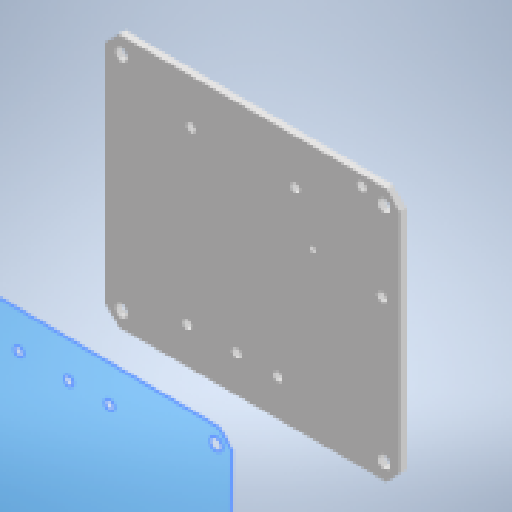
# Autodesk Inventor part: board_rpi
Saved by Autodesk Inventor 2025 (Build 290162000, 162)
## iProperties
Created: 2026-07-21
Part Number: board_rpi
Material: Типовые
Document SubType Name: Modeling
Designer: garin
Density: 1 g/cm^3
Appearance: По умолчанию
Author: garin
Autodesk Inventor part; units mm, degrees
ref_plane "YZ Plane" through (0, 0, 0) normal (1, 0, 0) x (0, 1, 0)
ref_plane "XZ Plane" through (0, 0, 0) normal (0, 1, 0) x (-1, 0, 0)
ref_plane "XY Plane" through (0, 0, 0) normal (0, 0, 1) x (1, 0, 0)
sketch "Эскиз1" plane through (0, 0, 0) normal (0, 0, 1) x (1, 0, 0)
  line L0 (-73.63, -2.23) -> (5.37, -2.23) projected
  arc A0 (5.37, -2.23) -> (8.37, 0.77) centre (5.37, 0.77) ccw projected
  line L1 (8.37, 0.77) -> (8.37, 50.77) projected
  arc A1 (8.37, 50.77) -> (5.37, 53.77) centre (5.37, 50.77) ccw projected
  line L2 (5.37, 53.77) -> (-73.63, 53.77) projected
  arc A2 (-73.63, 53.77) -> (-76.63, 50.77) centre (-73.63, 50.77) ccw projected
  line L3 (-76.63, 50.77) -> (-76.63, 0.77) projected
  arc A3 (-76.63, 0.77) -> (-73.63, -2.23) centre (-73.63, 0.77) ccw projected
  circle A4 centre (4.87, 50.27) radius 1.35 projected
  circle A5 centre (-53.13, 50.27) radius 1.35 projected
  circle A6 centre (0.07, 48.67) radius 0.325 projected
  circle A7 centre (-5.73, 48.67) radius 0.325 projected
  circle A8 centre (-68.88, 49.235) radius 1.65 projected
  circle A9 centre (4.87, 44.27) radius 1.55 projected
  circle A10 centre (-68.88, 37.805) radius 1.65 projected
  circle A11 centre (-53.13, 7.27) radius 1.55 projected
  circle A12 centre (4.87, 1.27) radius 1.35 projected
  circle A13 centre (-53.13, 1.27) radius 1.35 projected
  line L4 (5.37, -2.23) -> (8.37, -2.23) construction
  line L5 (8.37, -2.23) -> (8.37, 0.77) construction
  line L6 (8.37, 0.77) -> (5.37, 0.77) construction
  line L7 (5.37, 0.77) -> (5.37, -2.23) construction
  line L8 (8.37, -2.23) -> (-56.63, -2.23)
  line L9 (-56.63, -2.23) -> (-56.63, 53.77)
  line L10 (-56.63, 53.77) -> (8.37, 53.77)
  line L11 (8.37, 53.77) -> (8.37, -2.23)
  line L12 (8.37, -2.23) -> (-56.63, -2.23)
  line L13 (-56.63, -2.23) -> (-56.63, -13.23)
  line L14 (-56.63, -13.23) -> (8.37, -13.23)
  line L15 (8.37, -13.23) -> (8.37, -2.23)
  line L16 (-56.63, 53.77) -> (8.37, 53.77)
  line L17 (8.37, 53.77) -> (8.37, 61.77)
  line L18 (8.37, 61.77) -> (-56.63, 61.77)
  line L19 (-56.63, 61.77) -> (-56.63, 53.77)
  line L20 (0.1, 51.34) -> (-0.1, 51.34) construction
  line L21 (-0.1, 51.34) -> (-0.1, 51.74) construction
  line L22 (0.1, 51.74) -> (-0.1, 51.74) construction
  line L23 (0.1, 51.34) -> (0.1, 51.74) construction
  line L24 (0, 51.74) -> (0, 51.34) construction
  line L25 (0.1, 51.54) -> (-0.1, 51.54) construction
  circle A14 centre (0, 51.54) radius 1
  line L26 (4.5478, 32.4872) -> (4.3622, 32.4872) construction
  line L27 (4.3622, 32.4872) -> (4.3622, 32.6728) construction
  line L28 (4.3622, 32.6728) -> (4.5478, 32.6728) construction
  line L29 (4.5478, 32.6728) -> (4.5478, 32.4872) construction
  line L30 (4.455, 32.4872) -> (4.455, 32.6728) construction
  line L31 (4.5478, 32.58) -> (4.3622, 32.58) construction
  circle A15 centre (4.455, 32.58) radius 1
  line L32 (-37.8578, 43.7922) -> (-37.8578, 43.9778) construction
  line L33 (-37.8578, 43.9778) -> (-37.6722, 43.9778) construction
  line L34 (-37.6722, 43.9778) -> (-37.6722, 43.7922) construction
  line L35 (-37.6722, 43.7922) -> (-37.8578, 43.7922) construction
  line L36 (-37.765, 43.7922) -> (-37.765, 43.9778) construction
  line L37 (-37.6722, 43.885) -> (-37.8578, 43.885) construction
  circle A16 centre (-37.765, 43.885) radius 1
  line L38 (-14.8578, 43.7922) -> (-14.8578, 43.9778) construction
  line L39 (-14.8578, 43.9778) -> (-14.6722, 43.9778) construction
  line L40 (-14.6722, 43.9778) -> (-14.6722, 43.7922) construction
  line L41 (-14.6722, 43.7922) -> (-14.8578, 43.7922) construction
  line L42 (-14.765, 43.7922) -> (-14.765, 43.9778) construction
  line L43 (-14.6722, 43.885) -> (-14.8578, 43.885) construction
  circle A17 centre (-14.765, 43.885) radius 1
  circle A18 centre (-10.9214, 33.9778) radius 0.85 construction
  circle A19 centre (-10.9214, 33.9778) radius 0.6 projected
  line L44 (-18.88, 5.47) -> (-18.38, 5.47) construction
  line L45 (-18.88, 5.47) -> (-18.88, 6.22) construction
  line L46 (-18.88, 6.22) -> (-18.38, 6.22) construction
  line L47 (-18.38, 5.47) -> (-18.38, 6.22) construction
  line L48 (-27.88, 5.47) -> (-27.38, 5.47) construction
  line L49 (-27.88, 5.47) -> (-27.88, 6.22) construction
  line L50 (-27.88, 6.22) -> (-27.38, 6.22) construction
  line L51 (-27.38, 5.47) -> (-27.38, 6.22) construction
  line L52 (-38.88, 5.47) -> (-38.38, 5.47) construction
  line L53 (-38.88, 5.47) -> (-38.88, 6.22) construction
  line L54 (-38.88, 6.22) -> (-38.38, 6.22) construction
  line L55 (-38.38, 5.47) -> (-38.38, 6.22) construction
  line L56 (-18.38, 5.845) -> (-18.88, 5.845) construction
  line L57 (-18.63, 5.47) -> (-18.63, 6.22) construction
  circle A20 centre (-18.63, 5.845) radius 1
  line L58 (-27.38, 5.845) -> (-27.88, 5.845) construction
  line L59 (-27.63, 5.47) -> (-27.63, 6.22) construction
  line L60 (-38.38, 5.845) -> (-38.88, 5.845) construction
  line L61 (-38.63, 5.47) -> (-38.63, 6.22) construction
  circle A21 centre (-38.63, 5.845) radius 1
  circle A22 centre (-27.63, 5.845) radius 1
  point P0 (0, 0)
  point P1 (8.37, 0.77)
  point P2 (8.37, 53.77)
  dimension "d0" = 65
  dimension "d1" = 56
  dimension "d8" = 65
  dimension "d9" = 11
  dimension "d10" = 8
  dimension "d11" = 2
  dimension "d12" = 2
  dimension "d13" = 2
  dimension "d14" = 2
  dimension "d15" = 2
  dimension "d16" = 2
  dimension "d17" = 2
  constraints: 60 end point, 35 midpoint, 8 parallel, 7 centre point, 4 horizontal, 4 perpendicular
  measures "d0" distance of L9.end L10.end
  measures "d1" distance of L8.end L9.end
  measures "d8" distance of L14.end L13.end
  measures "d9" distance of L13.end L12.end
  measures "d10" distance of L17.end L16.end
  measures "d11" diameter of A14
  measures "d12" diameter of A15
  measures "d13" diameter of A16
  measures "d14" diameter of A17
  measures "d15" diameter of A20
  measures "d16" diameter of A21
  measures "d17" diameter of A22
extrude "Выдавливание1" add sketch "Эскиз1" along normal blind 1.5 contours L9 L2 A1 L1 A0 L0 | A0 L11 L8 | L10 L11 A1 | A6 | A7 | A9 | A11
chamfer "Фаска1" distance 3 angle 45 4 edges at (8.37, -2.23, 0.75) (8.37, 53.77, 0.75) (-56.63, 53.77, 0.75) (-56.63, -2.23, 0.75)
